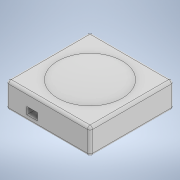
# Autodesk Inventor part: Button
Saved by Autodesk Inventor 2021 (Build 250183000, 183)
## iProperties
Created: 2021-05-27
Part Number: Button
Material: 一般
Document SubType Name: Modeling
Designer: gisen
Density: 1 g/cm^3
Appearance: 既定
Author: gisen
Autodesk Inventor part; units mm, degrees
ref_plane "YZ Plane" through (0, 0, 0) normal (1, 0, 0) x (0, 1, 0)
ref_plane "XZ Plane" through (0, 0, 0) normal (0, 1, 0) x (-1, 0, 0)
ref_plane "XY Plane" through (0, 0, 0) normal (0, 0, 1) x (1, 0, 0)
sketch "スケッチ1" plane through (0, 0, 0) normal (0, 1, 0) x (-1, 0, 0)
  line L0 (0, 0) -> (65, 0)
  line L1 (65, 0) -> (65, -65)
  line L2 (65, -65) -> (0, -65)
  line L3 (0, -65) -> (0, 0)
  dimension "d0" = 65
  dimension "d1" = 65
  constraints: 8 end point, 2 parallel, 1 horizontal, 1 perpendicular
  measures "d0" distance of L0.start L0.end
  measures "d1" distance of L0.end L1.end
extrude "押し出し1" add sketch "スケッチ1" along normal blind 20
sketch "スケッチ2" plane through (0, 20, 0) normal (0, 1, 0) x (1, 0, 0)
  line L0 (0, 65) -> (-65, 65) projected
  line L1 (-65, 65) -> (-65, 0) projected
  line L2 (-65, 0) -> (0, 0) projected
  line L3 (0, 0) -> (0, 65) projected
  circle A0 centre (-32.5, 32.5) radius 25
  dimension "d4" = 32.5
  dimension "d5" = 32.5
  dimension "d6" = 50
  constraints: 1 centre point
  measures "d4" distance from line of L2 A0.centre
  measures "d5" distance from line of L3 A0.centre
  measures "d6" diameter of A0
extrude "押し出し2" add sketch "スケッチ2" along normal blind 6 contours A0
ref_plane "作業平面1" through (-32.5, 0, 0) normal (1, 0, 0) x (0, 0, -1)
ref_plane "作業平面2" through (0, 10, 0) normal (0, 1, 0) x (1, 0, 0)
sketch "スケッチ3" plane through (-32.5, 0, 0) normal (1, 0, 0) x (0, 0, -1)
  line L0 (7.5, 20) -> (7.5, 26) projected
  line L1 (0, 20) -> (65, 20) projected
  line L2 (57.5, 26) -> (7.5, 26) projected
  line L3 (57.5, 26) -> (7.5, 26) projected
  line L4 (7.5, 20) -> (57.5, 20) projected
  line L5 (32.5, -55.0322) -> (32.5, 40.9092) projected
  arc A0 (32.5, 26) -> (7.5, 20) centre (35.4383, -41.3263) ccw
  point P0 (0, 0)
  point P1 (32.5, 26)
  constraints: 2 point on circle, 1 centre point, 1 midpoint, 1 point on line
revolve "回転1" cut sketch "スケッチ3" angle 360 about axis through (-32.5, 26, -32.5) along (0, 1, 0) contours L0 L2 A0
sketch "スケッチ7" plane through (-65, 0, 0) normal (0, 0, 1) x (1, 0, 0)
  line L0 (0, 0) -> (65, 0) projected
  line L1 (65, 0) -> (65, 20) projected
  line L2 (0, 20) -> (65, 20) projected
  line L3 (0, 0) -> (0, 20) projected
  line L4 (24.4, 4.4) -> (16, 4.4)
  line L5 (16, 4.4) -> (16, 10)
  line L6 (16, 10) -> (24.4, 10)
  line L7 (24.4, 10) -> (24.4, 4.4)
  dimension "d26" = 16
  dimension "d28" = 5.6
  dimension "d29" = 8.4
  dimension "d30" = 10
  constraints: 8 end point, 2 parallel, 1 horizontal, 1 perpendicular
  measures "d26" distance between parallel lines of L3 L5
  measures "d28" distance of L4.end L5.end
  measures "d29" distance of L5.end L6.end
  measures "d30" distance between parallel lines of L0 L6
extrude "押し出し4" cut sketch "スケッチ7" against normal blind 10 contours L4 L5 L6 L7
sketch "スケッチ5" plane through (0, 0, 0) normal (0, -1, 0) x (1, 0, 0)
  line L0 (0, -65) -> (-65, -65) projected
  line L1 (0, 0) -> (0, -65) projected
  line L2 (-65, 0) -> (0, 0) projected
  line L3 (-65, -65) -> (-65, 0) projected
  line L4 (-65, -65) -> (-65, 0) projected
  line L5 (-65, -32.5) -> (0, -32.5)
  line L6 (0, 0) -> (0, -65) projected
  point P0 (-12, -54)
  point P1 (-12, -11)
  dimension "d17" = 12
  dimension "d18" = 11
  constraints: 2 end point, 2 midpoint, 1 symmetric about line
  measures "d17" distance from line of L1 point (-12, -54)
  measures "d18" distance from line of L0 point (-12, -54)
fillet "フィレット1" radius 2 12 edges at (0, 10, 0) (0, 20, -32.5) (-32.5, 20, 0) (0, 0, -32.5) (-32.5, 0, 0) (0, 10, -65) (-32.5, 20, -65) (-32.5, 0, -65) (-65, 10, -65) (-65, 20, -32.5) (-65, 0, -32.5) (-65, 10, 0)
hole "穴1" at (-12, 0, -54) at (-12, 0, -11) direction (0, 1, 0) diameter 4.5 depth 10 tip angle 118
